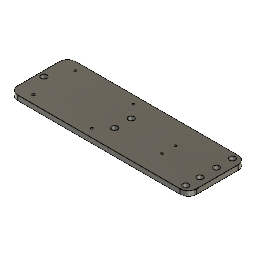
base v8 (Autodesk Fusion 360 design; units mm, degrees)
Autodesk Fusion 360 part; units mm, degrees
note: some values were not read from the file. Set by a fixed rule: which sketch regions a step uses.
sketch "Sketch1" plane through (0, 0, 0) normal (0, 0, 1) x (1, 0, 0)
  line L0 (10, 0) -> (205, 0)
  line L1 (215, 10) -> (215, 60)
  line L2 (205, 70) -> (10, 70)
  line L3 (0, 60) -> (0, 10)
  arc A0 (10, 70) -> (0, 60) centre (10, 60) ccw
  arc A1 (0, 10) -> (10, 0) centre (10, 10) ccw
  arc A2 (215, 60) -> (205, 70) centre (205, 60) ccw
  arc A3 (205, 0) -> (215, 10) centre (205, 10) ccw
  line L4 (205, 70) -> (205, 0)
  circle A4 centre (205, 43.9323) radius 3.5
  circle A5 centre (205, 23.9323) radius 3.5
  line L5 (102.5, 70) -> (102.5, 0)
  line L6 (205, 43.9323) -> (102.5, 43.9323)
  line L7 (205, 23.9323) -> (102.5, 23.9323)
  circle A6 centre (102.5, 43.9323) radius 3.5
  circle A7 centre (102.5, 23.9323) radius 3.5
  line L8 (89, 60) -> (49, 60)
  line L9 (49, 60) -> (49, 10)
  line L10 (49, 10) -> (89, 10)
  line L11 (89, 10) -> (89, 60)
  line L12 (102.5, 35) -> (89, 35)
  line L13 (49, 52.5466) -> (19, 52.5466)
  line L14 (19, 52.5466) -> (19, 17.4534)
  line L15 (19, 17.4534) -> (49, 17.4534)
  line L16 (49, 17.4534) -> (49, 52.5466)
  line L17 (19, 35) -> (49, 35)
  line L18 (0, 0) -> (0, 24.1752)
  line L19 (0, 0) -> (-15.0158, 0)
  line L20 (89, 60) -> (19, 60)
  line L21 (19, 60) -> (19, 10)
  line L22 (19, 10) -> (89, 10)
  line L23 (89, 10) -> (89, 60)
  circle A8 centre (89, 60) radius 1.25
  circle A9 centre (89, 10) radius 1.25
  circle A10 centre (19, 10) radius 1.5
  circle A11 centre (19, 60) radius 1.25
  point P0 (215, 0)
  point P1 (215, 70)
  point P2 (0, 70)
  dimension "d1" = 215
  dimension "d2" = 70
  dimension "d3" = 10
  dimension "d4" = 10
  dimension "d5" = 10
  dimension "d6" = 10
  dimension "d7" = 10
  dimension "d8" = 7
  dimension "d9" = 7
  dimension "d10" = 20
  dimension "d11" = 102.5
  dimension "d12" = 7
  dimension "d13" = 7
  dimension "d14" = 40
  dimension "d15" = 50
  dimension "d16" = 90
  dimension "d17" = 13.5
  dimension "d18" = 30
  dimension "d19" = 90
  dimension "d20" = 2.5
  dimension "d21" = 2.5
  dimension "d22" = 3
  dimension "d23" = 2.5
  constraint horizontal L0
  constraint vertical L1
  constraint horizontal L2
  constraint vertical L3
  constraint coincident P2 L2
  constraint coincident P2 L3
  constraint tangent L2 A0
  constraint tangent L3 A0
  constraint tangent L0 A1
  constraint tangent L3 A1
  constraint coincident P1 L1
  constraint coincident P1 L2
  constraint tangent L1 A2
  constraint tangent L2 A2
  constraint coincident P0 L0
  constraint coincident P0 L1
  constraint tangent L0 A3
  constraint tangent L1 A3
  constraint coincident L2 A2.end
  constraint coincident L0 A3.start
  constraint perpendicular L0 L4
  constraint coincident L4 A4.centre
  constraint coincident L4 A5.centre
  constraint coincident L2 L5.start
  constraint coincident L0 L5.end
  constraint perpendicular L0 L5
  constraint coincident A4.centre L6.start
  constraint coincident L5 L6.end
  constraint perpendicular L5 L6
  constraint coincident A5.centre L7.start
  constraint coincident L5 L7.end
  constraint perpendicular L5 L7
  constraint coincident L6.end A6.centre
  constraint coincident L7.end A7.centre
  constraint horizontal L8
  constraint vertical L9
  constraint horizontal L10
  constraint vertical L11
  constraint midpoint L5 L12.start
  constraint midpoint L11 L12.end
  constraint horizontal L13
  constraint vertical L14
  constraint horizontal L15
  constraint vertical L16
  constraint coincident L9 L13.start
  constraint midpoint L14 L17.start
  constraint midpoint L9 L17.end
  constraint coincident L18.start L19.start
  constraint vertical L18
  constraint perpendicular L18 L19
  constraint coincident L3 L18.end
  constraint horizontal L20
  constraint vertical L21
  constraint horizontal L22
  constraint vertical L23
  constraint collinear L14 L21
  constraint coincident L8.start L11.end
  constraint coincident L10.end L11.start
  constraint coincident L21.end L22.start
  constraint coincident L20.end L21.start
  measures "d1" distance of P1 P2
  measures "d2" distance of P0 P1
  measures "d3" radius of A0
  measures "d4" radius of A1
  measures "d5" radius of A2
  measures "d6" radius of A3
  measures "d7" distance of L1 L4
  measures "d8" diameter of A5
  measures "d9" diameter of A4
  measures "d10" distance of A4.centre A5.centre
  measures "d11" distance of L4 L5
  measures "d12" diameter of A6
  measures "d13" diameter of A7
  measures "d14" distance of L8.start L8.end
  measures "d15" distance of L8.start L10.end
  measures "d16" angle of L5 L12
  measures "d17" distance of L7.end L11
  measures "d18" distance of L13.start L13.end
  measures "d19" angle of L16 L17
  measures "d20" diameter of A8
  measures "d21" diameter of A9
  measures "d22" diameter of A10
  measures "d23" diameter of A11
extrude "Extrude1" add sketch "Sketch1" along normal blind 6 contours L0 L2 L3 A0 A1 L5 A6 A7 L18 | L0 L4 A5 L5 L7 A7 | L1 A2 A3 L4 A4 A5 | L4 A4 A5 L5 L6 L7 A6 A7 | L2 L4 A4 L5 L6 A6 | L8 L9 L10 L11 L16 L20 L22 L23 A8 A9 | L9 L13 L20 L21 A11 | L9 L13 L14 L16 L17 L21 | L9 L14 L15 L16 L17 L21 | L9 L15 L21 L22 A10
sketch "Sketch2" plane through (0, 0, 6) normal (0, 0, 1) x (-1, 0, 0)
  circle A0 centre (-19, -60) radius 1.25
  circle A1 centre (-102.5, -43.9323) radius 3.5
  circle A2 centre (-89, -60) radius 1.25
  circle A3 centre (-89, -10) radius 1.25
  circle A4 centre (-102.5, -23.9323) radius 3.5
  circle A5 centre (-19, -10) radius 1.5
  circle A6 centre (-205, -23.9323) radius 3.5
  circle A7 centre (-205, -43.9323) radius 3.5
  arc A8 (0, -10) -> (-10, 0) centre (-10, -10) ccw
  line L0 (-10, 0) -> (-205, 0)
  arc A9 (-205, 0) -> (-215, -10) centre (-205, -10) ccw
  line L1 (-215, -10) -> (-215, -60)
  arc A10 (-215, -60) -> (-205, -70) centre (-205, -60) ccw
  line L2 (-205, -70) -> (-10, -70)
  arc A11 (-10, -70) -> (0, -60) centre (-10, -60) ccw
  line L3 (0, -60) -> (0, -10)
  line L4 (-157.5, -70) -> (-157.5, 0)
  line L5 (-102.5, -43.9323) -> (-102.5, -23.9323)
  circle A12 centre (-157.5, -42.1823) radius 1.25
  circle A13 centre (-157.5, -25.6823) radius 1.25
  line L6 (-151.1278, -40.9323) -> (-166.7652, -40.9323)
  line L7 (-166.7652, -40.9323) -> (-166.7652, -26.9323)
  line L8 (-166.7652, -26.9323) -> (-151.1278, -26.9323)
  line L9 (-151.1278, -26.9323) -> (-151.1278, -40.9323)
  line L10 (-151.1278, -33.9323) -> (-102.5, -33.9323)
  dimension "d26" = 55
  dimension "d27" = 14
  dimension "d28" = 90
  dimension "d29" = 2.5
  dimension "d30" = 2.5
  constraint coincident L2 L4.start
  constraint coincident L0 L4.end
  constraint perpendicular L0 L4
  constraint coincident A1.centre L5.start
  constraint coincident A4.centre L5.end
  constraint coincident L4 A12.centre
  constraint coincident L4 A13.centre
  constraint horizontal L6
  constraint vertical L7
  constraint horizontal L8
  constraint vertical L9
  constraint tangent A12 L6
  constraint tangent A13 L8
  constraint midpoint L9 L10.start
  constraint midpoint L5 L10.end
  measures "d26" distance of L4 L5
  measures "d27" distance of L6.end L7.end
  measures "d28" angle of L5 L10
  measures "d29" diameter of A12
  measures "d30" diameter of A13
extrude "Extrude2" cut sketch "Sketch2" against normal blind 5 contours L4 A13 | L4 A13 | L4 A12 | L4 A12
sketch "Sketch3" plane through (0, 0, 6) normal (0, 0, 1) x (-1, 0, 0)
  circle A0 centre (-157.5, -42.1823) radius 1.25
  circle A1 centre (-157.5, -25.6823) radius 1.25
  circle A2 centre (-205, -43.9323) radius 3.5
  circle A3 centre (-19, -10) radius 1.5
  circle A4 centre (-89, -60) radius 1.25
  circle A5 centre (-89, -10) radius 1.25
  circle A6 centre (-102.5, -43.9323) radius 3.5
  circle A7 centre (-19, -60) radius 1.25
  circle A8 centre (-205, -23.9323) radius 3.5
  circle A9 centre (-102.5, -23.9323) radius 3.5
  arc A10 (0, -10) -> (-10, 0) centre (-10, -10) ccw
  line L0 (-10, 0) -> (-205, 0)
  arc A11 (-205, 0) -> (-215, -10) centre (-205, -10) ccw
  line L1 (-215, -10) -> (-215, -60)
  arc A12 (-215, -60) -> (-205, -70) centre (-205, -60) ccw
  line L2 (-205, -70) -> (-10, -70)
  arc A13 (-10, -70) -> (0, -60) centre (-10, -60) ccw
  line L3 (0, -60) -> (0, -10)
  line L4 (-6.5, -60) -> (-6.5, -10)
  circle A14 centre (-6.5, -35) radius 3.5
  line L5 (-10, -60) -> (-10, -10)
  line L6 (-6.5, -35) -> (0, -35)
  line L7 (-205, -70) -> (-205, 0)
  circle A15 centre (-205, -63) radius 3.5
  circle A16 centre (-205, -7) radius 3.5
  dimension "d33" = 7
  dimension "d36" = 7
  dimension "d37" = 7
  dimension "d38" = 7
  dimension "d39" = 7
  constraint perpendicular L0 L4
  constraint midpoint L4 A14.centre
  constraint coincident A13.centre L5.start
  constraint coincident A10.centre L5.end
  constraint tangent A14 L5
  constraint coincident A14.centre L6.start
  constraint midpoint L3 L6.end
  constraint perpendicular L3 L6
  constraint coincident L2 A12.end
  constraint coincident L0 A11.start
  constraint perpendicular L0 L7
  constraint coincident L7 A15.centre
  constraint coincident L7 A16.centre
  constraint coincident A2.centre L7
  measures "d33" diameter of A14
  measures "d36" diameter of A15
  measures "d37" diameter of A16
  measures "d38" distance of L2 A15.centre
  measures "d39" distance of L0 A16.centre
extrude "Extrude3" cut sketch "Sketch3" against normal blind 7 contours L7 A15 | L7 A15 | L7 A16 | L7 A16 | L4 A14 | L4 A14 L6 | L4 A14 L6
extrude "Extrude4" cut 1 faces at (157.8221, 41.8565, 1) along direction (0, 0, -1) blind 5
extrude "Extrude5" cut 1 faces at (157.1946, 25.2747, 1) along direction (0, 0, -1) blind 5
